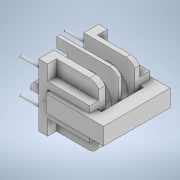
# Autodesk Inventor part: UU10.5
Saved by Autodesk Inventor 2020 (Build 240168000, 168)
## iProperties
Created: 2021-07-21
Part Number: UU10.5
Material: Типовые
Document SubType Name: Modeling
Designer: VB
Density: 1 g/cm^3
Appearance: По умолчанию
Author: VB
Autodesk Inventor part; units mm, degrees
ref_plane "YZ Plane" through (0, 0, 0) normal (1, 0, 0) x (0, 1, 0)
ref_plane "XZ Plane" through (0, 0, 0) normal (0, 1, 0) x (-1, 0, 0)
ref_plane "XY Plane" through (0, 0, 0) normal (0, 0, 1) x (1, 0, 0)
sketch "Эскиз1" plane through (0, 0, 0) normal (0, 1, 0) x (-1, 0, 0)
  line L0 (9, 8.8) -> (9, -8.8) construction
  line L1 (-9, -8.8) -> (-9, 8.8) construction
  line L2 (-9, 8.8) -> (9, -8.8) construction
  line L3 (9, 8.8) -> (-9, -8.8) construction
  line L4 (9, 0) -> (9, 0.5)
  line L5 (9, 0.5) -> (-9, 0.5)
  line L6 (9, 0) -> (9, -0.4719)
  line L7 (9, -0.4719) -> (-9, -0.4719)
  line L8 (-9, 0.5) -> (-9, -0.4719)
  line L9 (9, 0) -> (9, 4.3404) construction
  line L10 (9, 0) -> (9, -4.4046) construction
  line L11 (9, 4.3404) -> (-9, 4.3404)
  line L12 (-9, 4.3404) -> (-9, 8.8)
  line L13 (-9, 8.8) -> (9, 8.8)
  line L14 (9, 8.8) -> (9, 4.3404)
  line L15 (9, -4.4046) -> (-9, -4.4046)
  line L16 (-9, -4.4046) -> (-9, -8.8)
  line L17 (-9, -8.8) -> (9, -8.8)
  line L18 (9, -8.8) -> (9, -4.4046)
  point P0 (0, 0)
  dimension "d0" = 18
  dimension "d1" = 17.6
  dimension "d2" = 0.5
  constraints: 38 end point, 6 point on line, 5 parallel, 4 perpendicular, 3 midpoint, 2 horizontal, 1 collinear
  measures "d0" distance of L0.end L1.start
  measures "d1" distance of L0.start L0.end
  measures "d2" distance of L4.start L4.end
extrude "Выдавливание1" add sketch "Эскиз1" along normal blind 18.4
sketch "Эскиз4" plane through (9, 0, 8.8) normal (1, 0, 0) x (0, 0, -1)
  line L0 (13.2046, 0) -> (17.6, 0) projected
  line L1 (14.5773, 0) -> (21.0298, 0)
  line L2 (21.0298, 0) -> (21.0298, 4.45)
  line L3 (21.0298, 4.45) -> (14.5773, 4.45)
  line L4 (14.5773, 4.45) -> (14.5773, 0)
  line L5 (14.5773, 18.4) -> (21.6, 18.4)
  line L6 (21.6, 18.4) -> (21.6, 13.95)
  line L7 (21.6, 13.95) -> (14.5773, 13.95)
  line L8 (14.5773, 13.95) -> (14.5773, 18.4)
  line L9 (4.4596, 18.4) -> (0, 18.4) projected
  line L10 (2.5726, 18.4) -> (-5.1704, 18.4)
  line L11 (-5.1704, 18.4) -> (-5.1704, 13.95)
  line L12 (-5.1704, 13.95) -> (2.5726, 13.95)
  line L13 (2.5726, 13.95) -> (2.5726, 18.4)
  line L14 (4.4596, 0) -> (0, 0) projected
  line L15 (2.5726, 0) -> (-6.491, 0)
  line L16 (-6.491, 0) -> (-6.491, 4.45)
  line L17 (-6.491, 4.45) -> (2.5726, 4.45)
  line L18 (2.5726, 4.45) -> (2.5726, 0)
  line L19 (20.6227, 11.95) -> (14.5773, 11.95)
  line L20 (14.5773, 11.95) -> (14.5773, 6.45)
  line L21 (14.5773, 6.45) -> (20.6227, 6.45)
  line L22 (20.6227, 6.45) -> (20.6227, 11.95)
  line L23 (17.6, 0) -> (17.6, 18.4) projected
  line L24 (20.6227, 11.95) -> (14.5773, 6.45) construction
  line L25 (14.5773, 11.95) -> (20.6227, 6.45) construction
  line L26 (-2.5726, 11.95) -> (2.5726, 11.95)
  line L27 (2.5726, 11.95) -> (2.5726, 6.45)
  line L28 (2.5726, 6.45) -> (-2.5726, 6.45)
  line L29 (-2.5726, 6.45) -> (-2.5726, 11.95)
  line L30 (0, 0) -> (0, 18.4) projected
  line L31 (-2.5726, 11.95) -> (2.5726, 6.45) construction
  line L32 (2.5726, 11.95) -> (-2.5726, 6.45) construction
  point P0 (8.8, 0)
  point P1 (17.6, 9.2)
  point P2 (0, 9.2)
  dimension "d12" = 5.5
  dimension "d41" = 2
  dimension "d42" = 2
  dimension "d43" = 2
  constraints: 56 end point, 12 parallel, 6 horizontal, 6 midpoint, 6 perpendicular, 5 point on line
  measures "d12" distance of L20.end L19.end
  measures "d41" distance between parallel lines of L12 L26
  measures "d42" distance between parallel lines of L17 L28
  measures "d43" distance between parallel lines of L21 L3
extrude "Выдавливание2" cut sketch "Эскиз4" against normal blind 12.4
sketch "Эскиз6" plane through (9, 0, 4.3404) normal (0, 0, -1) x (-1, 0, 0)
  line L0 (9, 0) -> (9, 18.4) construction
  line L1 (18, 18.4) -> (0, 18.4) projected
  line L2 (9, 9.2) -> (7.5, 9.2) construction
  circle A0 centre (7.5, 9.2) radius 5.5
  dimension "d16" = 1.5
  dimension "d53" = 11
  constraints: 4 end point, 2 midpoint, 1 centre point, 1 coincident, 1 horizontal
  measures "d16" distance of L2.start L2.end
  measures "d53" diameter of A0
sketch "Эскиз7" plane through (-9, 0, -8.8) normal (0, 0, -1) x (-1, 0, 0)
  line L0 (-18, 13.95) -> (-5.6, 13.95) projected
  line L1 (-18, 0) -> (-18, 18.4) construction
  line L2 (-21, -3) -> (-15, -3) construction
  line L3 (-15, -3) -> (-15, 3) construction
  line L4 (-15, 3) -> (-21, 3) construction
  line L5 (-21, 3) -> (-21, -3) construction
  line L6 (-21, -3) -> (-15, 3) construction
  line L7 (-15, -3) -> (-21, 3) construction
  line L8 (-21.3737, 21.4) -> (-15.3737, 21.4) construction
  line L9 (-15.3737, 21.4) -> (-15.3737, 15.4) construction
  line L10 (-15.3737, 15.4) -> (-21.3737, 15.4) construction
  line L11 (-21.3737, 15.4) -> (-21.3737, 21.4) construction
  line L12 (-21.3737, 21.4) -> (-15.3737, 15.4) construction
  line L13 (-15.3737, 21.4) -> (-21.3737, 15.4) construction
  arc A0 (-18, 3) -> (-15, 0) centre (-15, 3) ccw
  arc A1 (-15.3737, 18.4) -> (-18, 13.95) centre (-15.3737, 15.4) ccw
  line L14 (-18, 3) -> (-18, 0)
  line L15 (-15, 0) -> (-18, 0)
  line L16 (-15.3737, 18.4) -> (-18, 18.4)
  line L17 (-18, 13.95) -> (-18, 18.4)
  point P0 (-9, 0)
  dimension "d21" = 6
  dimension "d22" = 6
  constraints: 32 end point, 5 midpoint, 5 parallel, 4 point on circle, 3 perpendicular, 2 centre point, 2 coincident, 2 horizontal, 2 tangent, 1 collinear
  measures "d21" distance of L3.end L2.end
  measures "d22" distance of L8.end L9.end
extrude "Выдавливание3" add sketch "Эскиз6" along normal up to surface (8.745 mm away)
extrude "Выдавливание4" cut sketch "Эскиз7" against normal blind 23
ref_plane "РабПлоскость1" through (-3.4, 9.2, 8.8) normal (0, -1, 0) x (0, 0, -1)
sketch "Эскиз9" plane through (-3.4, 9.2, 8.8) normal (0, -1, 0) x (0, 0, -1)
  line L0 (-0.964, 17.4) -> (18.536, 17.4)
  line L1 (18.536, 17.4) -> (18.536, 0.5)
  line L2 (18.536, 0.5) -> (-0.964, 0.5)
  line L3 (-0.964, 0.5) -> (-0.964, 17.4)
  line L4 (2.3726, 13.4) -> (14.7773, 13.4)
  line L5 (14.7773, 13.4) -> (14.7773, 4.5)
  line L6 (14.7773, 4.5) -> (2.3726, 4.5)
  line L7 (2.3726, 4.5) -> (2.3726, 13.4)
  line L8 (8.786, 13.2041) -> (8.786, 18.9436) construction
  line L9 (0, 0) -> (0, 12.4) projected
  line L10 (17.6, -5.6) -> (13.2046, -5.6) projected
  point P0 (8.8, 3.4)
  point P1 (17.6, 0)
  point P2 (2.5726, 12.4)
  point P3 (14.5773, 12.4)
  dimension "d30" = 8.786
  dimension "d31" = 9.75
  dimension "d32" = 9.75
  dimension "d33" = 23
  dimension "d34" = 0.5
  dimension "d35" = 0.2
  dimension "d36" = 0.2
  dimension "d37" = 4
  dimension "d38" = 4
  constraints: 18 end point, 4 parallel, 2 horizontal, 2 perpendicular, 1 vertical
  measures "d30" distance between parallel lines of L9 L8
  measures "d31" distance between parallel lines of L3 L8
  measures "d32" distance between parallel lines of L1 L8
  measures "d33" distance between parallel lines of L0 L10
  measures "d34" distance from line of point (17.6, 0) L2
  measures "d35" distance from line of point (2.573, 12.4) L7
  measures "d36" distance from line of point (14.577, 12.4) L5
  measures "d37" distance between parallel lines of L0 L4
  measures "d38" distance between parallel lines of L2 L6
extrude "Выдавливание5" add sketch "Эскиз9" along normal mid plane 5
sketch "Эскиз10" plane through (-9, 0, 4.3404) normal (-1, 0, 0) x (0, 0, 1)
  line L0 (4.4596, 6.45) -> (4.4596, 11.95) projected
  line L1 (4.4596, 9.2) -> (-13.9375, 9.2) construction
  line L2 (-14.0763, 6.7) -> (-14.0763, 11.7) projected
  line L3 (1, 9.2) -> (2.9596, 9.2) construction
  line L4 (1, 8.2) -> (2.9596, 8.2)
  line L5 (2.9596, 10.2) -> (1, 10.2)
  arc A0 (1, 10.2) -> (1, 8.2) centre (1, 9.2) ccw
  arc A1 (2.9596, 8.2) -> (2.9596, 10.2) centre (2.9596, 9.2) ccw
  line L6 (0, 0) -> (0, 18.4) projected
  line L7 (4.4596, 0) -> (4.4596, 18.4) projected
  line L8 (-9.745, 9.2) -> (-11.6404, 9.2) construction
  line L9 (-9.745, 10.2) -> (-11.6404, 10.2)
  line L10 (-11.6404, 8.2) -> (-9.745, 8.2)
  arc A2 (-9.745, 8.2) -> (-9.745, 10.2) centre (-9.745, 9.2) ccw
  arc A3 (-11.6404, 10.2) -> (-11.6404, 8.2) centre (-11.6404, 9.2) ccw
  line L11 (-8.745, 0) -> (-8.745, 18.4) projected
  line L12 (-13.1404, 0) -> (-13.1404, 18.4) projected
  line L13 (-4.8123, 0) -> (-4.8123, 18.4) projected
  line L14 (-3.8404, 0) -> (-3.8404, 3) projected
  line L15 (-4.8123, 0) -> (-3.8404, 0)
  line L16 (-3.8404, 0) -> (-3.8404, 3)
  line L17 (-3.8404, 3) -> (-4.8123, 3)
  line L18 (-4.8123, 3) -> (-4.8123, 0)
  line L19 (-4.8123, 3) -> (-4.8123, 16.85) projected
  line L20 (-3.8404, 18.4) -> (-4.8123, 18.4)
  line L21 (-4.8123, 18.4) -> (-4.8123, 15.4)
  line L22 (-4.8123, 15.4) -> (-3.8404, 15.4)
  line L23 (-3.8404, 15.4) -> (-3.8404, 18.4)
  line L24 (8.1135, -3.7823) -> (-17.89, -3.7823)
  line L25 (-17.89, -3.7823) -> (-17.89, 22.1054)
  line L26 (-17.89, 22.1054) -> (8.1135, 22.1054)
  line L27 (8.1135, 22.1054) -> (8.1135, -3.7823)
  point P0 (-4.3404, 0)
  point P1 (1.9798, 9.2)
  point P2 (-10.6927, 9.2)
  point P3 (-4.8123, 3)
  dimension "d44" = 2
  dimension "d45" = 1
  dimension "d46" = 1.5
  dimension "d47" = 1
  dimension "d48" = 1.5
  dimension "d49" = 3
  dimension "d50" = 3
  constraints: 42 end point, 8 parallel, 8 point on circle, 8 tangent, 5 point on line, 4 centre point, 4 perpendicular, 3 horizontal, 3 midpoint
  measures "d44" diameter of A1
  measures "d45" distance from line of L6 L3.start
  measures "d46" distance from line of L7 L3.end
  measures "d47" distance from line of L11 L8.start
  measures "d48" distance from line of L12 L8.end
  measures "d49" distance of L14.end L15.end
  measures "d50" distance of L21.end L20.end
extrude "Выдавливание6" cut sketch "Эскиз10" against normal blind 3
sketch "Эскиз11" plane through (-6, 0, 4.3404) normal (-1, 0, 0) x (0, 0, 1)
  line L0 (-4.3263, -2.8057) -> (-4.3263, 20.2349) construction
  line L1 (5.7896, 9.2) -> (-19.3839, 9.2) construction
  line L2 (2.1737, 14.2) -> (-10.8263, 14.2) construction
  line L3 (-10.8263, 14.2) -> (-10.8263, 4.2) construction
  line L4 (-10.8263, 4.2) -> (2.1737, 4.2) construction
  line L5 (2.1737, 4.2) -> (2.1737, 14.2) construction
  line L6 (2.1737, 14.2) -> (-10.8263, 4.2) construction
  line L7 (-10.8263, 14.2) -> (2.1737, 4.2) construction
  circle A0 centre (2.1737, 4.2) radius 0.35
  circle A1 centre (-10.8263, 4.2) radius 0.35
  circle A2 centre (-10.8263, 14.2) radius 0.35
  circle A3 centre (2.1737, 14.2) radius 0.35
  point P0 (-4.3404, 0)
  point P1 (-4.3263, 9.2)
  dimension "d54" = 13
  dimension "d55" = 10
  dimension "d56" = 0.7
  dimension "d57" = 0.7
  dimension "d58" = 0.7
  dimension "d59" = 0.7
  constraints: 16 end point, 4 centre point, 4 coincident, 2 horizontal, 2 midpoint, 2 parallel, 2 point on line, 1 perpendicular, 1 vertical
  measures "d54" distance of L4.end L3.end
  measures "d55" distance of L3.end L2.end
  measures "d56" diameter of A0
  measures "d57" diameter of A1
  measures "d58" diameter of A2
  measures "d59" diameter of A3
extrude "Выдавливание7" add sketch "Эскиз11" along normal blind 7.5
